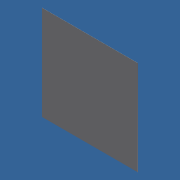
# Autodesk Inventor part: COMMON
Saved by Autodesk Inventor 2015 SP1 (Build 190203100, 203)
## iProperties
Created: 2015-08-21
Material: Generic
Vendor: DIGIKEY
Document SubType Name: Modeling
Designer: NEGRASHOVI
Density: 1 g/cm^3
Appearance: Default
Project: COMMON
Description: THERMAL PAD
Part Number: COMMON
RuleStatus: InUse
AfterDocSave0: file://Part Number Cleaner
LAB/DEPT: COMMON
REQUESTING SCIENTIST: COMMON
SURFACE ROUGHNESS: N/A
DESIGN DEPARTMENT: HHMI: JRC - ID&F
SPECIAL FINISH: NONE
ALTERED ITEM PART NUMBER: N/A
ALTERED ITEM VENDOR: N/A
ALTERED ITEM DESCRIPTION: N/A
Author: NEGRASHOVI
Revision Number: -
Autodesk Inventor part; units mm, degrees
ref_plane "YZ Plane" through (0, 0, 0) normal (1, 0, 0) x (0, 1, 0)
ref_plane "XZ Plane" through (0, 0, 0) normal (0, 1, 0) x (-1, 0, 0)
ref_plane "XY Plane" through (0, 0, 0) normal (0, 0, 1) x (1, 0, 0)
sketch "Sketch1" plane through (0, 0, 0) normal (0, 0, 1) x (1, 0, 0)
  line L0 (-77.216, -76.2) -> (77.216, -76.2)
  line L1 (77.216, -76.2) -> (77.216, 76.2)
  line L2 (77.216, 76.2) -> (-77.216, 76.2)
  line L3 (-77.216, 76.2) -> (-77.216, -76.2)
  point P0 (0, 0)
  point P1 (77.216, 0)
  point P2 (0, 76.2)
  dimension "d0" = 154.432
  dimension "d1" = 152.4
  constraints: 8 end point, 2 midpoint, 2 parallel, 1 horizontal, 1 horizontal alignment, 1 perpendicular, 1 vertical alignment
  measures "d0" distance of L1.end L2.end
  measures "d1" distance of L0.end L1.end
extrude "Extrusion1" add sketch "Sketch1" along normal blind 0.254
body "Solid1"
